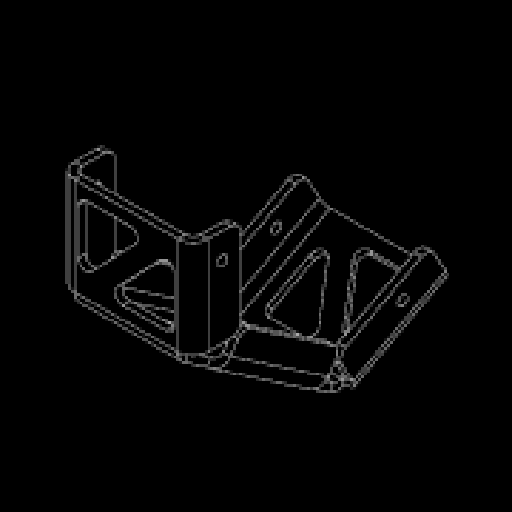
# Autodesk Inventor part: HipCoverTop
Saved by Autodesk Inventor 2025.2 (Build 292293000, 293)
## iProperties
Created: 2020-05-24
Part Number: HipCoverTop
Material: Generic
Document SubType Name: Sheet Metal
Designer: valer
Density: 1 g/cm^3
Sheet Metal Rule: Default
Appearance: Default
Author: valer
Autodesk Inventor part; units mm, degrees
ref_plane "YZ Plane" through (0, 0, 0) normal (1, 0, 0) x (0, 1, 0)
ref_plane "XZ Plane" through (0, 0, 0) normal (0, 1, 0) x (-1, 0, 0)
ref_plane "XY Plane" through (0, 0, 0) normal (0, 0, 1) x (1, 0, 0)
sketch "Base" plane through (0, 0, 0) normal (0, 0, 1) x (1, 0, 0)
  line L0 (0, 0) -> (44.58, 0)
  line L1 (44.58, 0) -> (44.58, -65.2018)
  line L2 (44.58, -65.2018) -> (0, -65.2018)
  line L3 (0, -65.2018) -> (0, 0)
  dimension "d0" = 65.2018
  dimension "d1" = 44.58
  measures "d0" distance of L2.end L0.start
  measures "d1" distance of L0.start L0.end
extrude "Plate1" add sketch "Base" along normal blind 5
sketch "Sketch2" plane through (5, 0, 5) normal (-1, 0, 0) x (0, -1, 0)
  line L0 (65.2018, 0) -> (0, 0)
  line L1 (0, 0) -> (0, -31.75)
  line L2 (0, -31.75) -> (65.2018, -31.75)
  line L3 (65.2018, -31.75) -> (65.2018, 0)
  constraints: 6 end point, 1 horizontal, 1 perpendicular, 1 vertical
edge flange "MountFeature" height 31.75 angle 90 thickness 5 bend radius 5 thickness toward (-1, 0, 0) relief straight relief width 5 relief depth 2.5 edges at (0, -32.6009, 0) wall of the first edge with corners at (5, -65.2018, 5) (5, 0, 5) (5, 0, -26.75) (5, -65.2018, -26.75)
bend "Bend1"
corner "Corner1"
mirror "MirrorFeature" about plane through (44.58, 0, 0) normal (1, 0, 0)
sketch "GenerativeCut1" plane through (0, 0, 5) normal (0, 0, 1) x (1, 0, 0)
  line L0 (12.7, -8.4667) -> (12.7, -56.7351)
  line L1 (12.7, -56.7351) -> (58.8832, -8.4667)
  line L2 (58.8832, -8.4667) -> (12.7, -8.4667)
  line L3 (79.16, 0) -> (10, 0) projected
  line L4 (30.2768, -56.7351) -> (76.46, -8.4667)
  line L5 (76.46, -8.4667) -> (76.46, -56.7351)
  line L6 (76.46, -56.7351) -> (30.2768, -56.7351)
  line L7 (58.8832, -8.4667) -> (76.46, -8.4667) construction
  line L8 (12.7, -56.7351) -> (30.2768, -56.7351) construction
  line L9 (0, -65.2018) -> (0, 0) projected
  line L10 (89.16, -65.2018) -> (89.16, 0) projected
  line L11 (79.16, -65.2018) -> (10, -65.2018) projected
  dimension "d23" = 8.4667
  dimension "d24" = 12.7
  dimension "d25" = 12.7
  dimension "d26" = 8.4667
  dimension "d27" = 12.7
  constraints: 16 end point, 2 parallel, 2 perpendicular, 1 collinear, 1 horizontal, 1 vertical
  measures "d23" distance between parallel lines of L3 L2
  measures "d24" distance between parallel lines of L9 L0
  measures "d25" distance between parallel lines of L5 L10
  measures "d26" distance between parallel lines of L11 L6
  measures "d27" distance between parallel lines of L4 L1
extrude "GenerativeCut1Feature" cut sketch "GenerativeCut1" against normal blind 25.4
fillet "GenerativeCut1FilletsFeature" radius 5.08 6 edges at (12.7, -8.4667, 2.5) (12.7, -56.7351, 2.5) (58.8832, -8.4667, 2.5) (76.46, -8.4667, 2.5) (30.2768, -56.7351, 2.5) (76.46, -56.7351, 2.5)
sketch "Sketch5" plane through (79.16, -69.3397, -2.1932) normal (0, -0.8275708, 0.5613614) x (1, 0, 0)
  line L0 (-69.16, 0) -> (0, 0)
  line L1 (0, 0) -> (0, 116.6197)
  line L2 (0, 116.6197) -> (-69.16, 116.6197)
  line L3 (-69.16, 116.6197) -> (-69.16, 0)
  constraints: 6 end point, 1 horizontal, 1 perpendicular, 1 vertical
edge flange "KneeFlangeFeature" height 121.92 angle 55.85 thickness 5 bend radius 5 thickness toward (0, -0.8275708, 0.5613614) relief straight relief width 5 relief depth 2.5 edges at (44.58, -65.2018, 5) wall of the first edge with corners at (10, -69.3397, -2.1932) (79.16, -69.3397, -2.1932) (79.16, -134.8054, -98.7042) (10, -134.8054, -98.7042)
bend "Bend2"
corner "Corner2"
sketch "Sketch6" plane through (10, -135.0807, -103.8615) normal (0, -0.8826196, -0.4700879) x (1, 0, 0)
  line L0 (69.16, 0) -> (0, 0)
  line L1 (0, 0) -> (0, -70.1688)
  line L2 (0, -70.1688) -> (69.16, -70.1688)
  line L3 (69.16, -70.1688) -> (69.16, 0)
  constraints: 6 end point, 1 horizontal, 1 perpendicular, 1 vertical
edge flange "KneeBottomFlangeFeature" height 76.2 angle 62.19 thickness 5 bend radius 5 thickness toward (0, -0.8826196, -0.4700879) relief straight relief width 5 relief depth 2.5 edges at (44.58, -134.8054, -98.7042) wall of the first edge with corners at (79.16, -135.0807, -103.8615) (10, -135.0807, -103.8615) (10, -102.0952, -165.7938) (79.16, -102.0952, -165.7938)
bend "Bend3"
corner "Corner3"
sketch "Sketch8" plane through (5, -130.6676, -101.511) normal (-1, 0, 0) x (0, -1, 0)
  line L0 (-32.9855, -61.9324) -> (0, 0)
  line L1 (0, 0) -> (-19.197, 10.2244)
  line L2 (-19.197, 10.2244) -> (-52.1825, -51.708)
  line L3 (-52.1825, -51.708) -> (-32.9855, -61.9324)
  constraints: 6 end point, 1 perpendicular, 2 other
edge flange "KneeBottomSidesFeature" height 31.75 angle 90 thickness 5 bend radius 5 thickness toward (-1, 0, 0) relief straight relief width 5 relief depth 2.5 corner gap 5 corner form 0 edges at (10, -118.5879, -134.8277) (79.16, -118.5879, -134.8277) wall of the first edge with corners at (5, -97.6821, -163.4434) (5, -130.6676, -101.511) (5, -111.4706, -91.2866) (5, -78.4851, -153.219)
bend "Bend4"
corner "Corner4"
fillet "OutsideFilletsFeature" radius 6.35 8 edges at (2.5, -65.2018, -26.75) (2.5, 0, -26.75) (2.5, -111.4706, -91.2866) (86.66, -78.4851, -153.219) (2.5, -78.4851, -153.219) (86.66, -111.4706, -91.2866) (86.66, -65.2018, -26.75) (86.66, 0, -26.75)
sketch "Sketch10" plane through (10, -73.4775, 0.6136) normal (0, -0.8275708, 0.5613614) x (1, 0, 0)
  line L0 (-5, -15.5299) -> (-10, -15.5299) projected
  line L1 (-5, -99.6109) -> (-10, -99.6109) projected
  line L2 (-10, -18.0699) -> (0, -18.0699)
  line L3 (0, -18.0699) -> (0, -97.0709)
  line L4 (0, -97.0709) -> (-10, -97.0709)
  line L5 (-10, -97.0709) -> (-10, -18.0699)
  line L6 (-10, 0) -> (-10, -12.7446) projected
  line L7 (0, 0) -> (0, -116.6197) projected
  point P0 (-10, 40.7396)
  dimension "d65" = 2.54
  dimension "d66" = 2.54
  constraints: 8 end point, 2 collinear, 2 parallel, 1 horizontal, 1 perpendicular
  measures "d65" distance between parallel lines of L0 L2
  measures "d66" distance between parallel lines of L1 L4
sheet face with bend "SideFlangeBaseFeature" sketch "Sketch10" thickness 5 toward (0, 0.8275708, -0.5613614) bend radius 5 relief straight relief width 5 relief depth 2.5
bend "Bend5"
sketch "Sketch11" plane through (5, -83.6213, -14.3405) normal (-1, 0, 0) x (0, -1, 0)
  line L0 (44.3481, -65.3789) -> (0, 0)
  line L1 (0, 0) -> (-21.0203, -14.2586)
  line L2 (-21.0203, -14.2586) -> (23.3278, -79.6375)
  line L3 (23.3278, -79.6375) -> (44.3481, -65.3789)
  constraints: 6 end point, 1 perpendicular, 2 other
edge flange "SideFlangeFeature" height 25.4 angle 90 thickness 5 bend radius 5 thickness toward (-1, 0, 0) relief straight relief width 5 relief depth 2.5 edges at (0, -101.6575, -49.8368) wall of the first edge with corners at (5, -127.9694, -79.7194) (5, -83.6213, -14.3405) (5, -62.601, -28.5991) (5, -106.9491, -93.978)
bend "Bend6"
corner "Corner5"
ref_plane "MiddlePlane" through (44.58, -97.6821, -163.4434) normal (-1, 0, 0) x (0, -0.4700879, 0.8826196)
mirror "SideFlangeMirrorFeature" about plane through (44.58, -97.6821, -163.4434) normal (-1, 0, 0) of "SideFlangeFeature"
fillet "SideFlangeFilletsFeature" radius 6.35 4 edges at (2.5, -106.9491, -93.978) (86.66, -106.9491, -93.978) (2.5, -62.601, -28.5991) (86.66, -62.601, -28.5991)
sketch "Rais" plane through (10, -73.4775, 0.6136) normal (0, -0.8275708, 0.5613614) x (1, 0, 0)
  line L0 (69.16, 0) -> (0, 0) construction
  line L1 (0, -116.6197) -> (69.16, -116.6197) construction
  line L2 (0, 0) -> (69.16, 0) construction
  line L3 (34.58, 0) -> (34.58, -116.6197) construction
  line L4 (0, -116.6197) -> (69.16, -116.6197) construction
  line L5 (26.3701, -42.5901) -> (17.3899, -33.6099) construction
  line L6 (24.1251, -44.8352) -> (15.1448, -35.8549)
  line L7 (19.6349, -31.3648) -> (28.6152, -40.3451)
  arc A0 (24.1251, -44.8352) -> (28.6152, -40.3451) centre (26.3701, -42.5901) ccw
  arc A1 (19.6349, -31.3648) -> (15.1448, -35.8549) centre (17.3899, -33.6099) ccw
  line L8 (0, -18.0699) -> (0, -97.0709) construction
  line L9 (0, -57.5704) -> (69.16, -57.5704) construction
  line L10 (69.16, -97.0709) -> (69.16, -18.0699) construction
  line L11 (45.0349, -44.8352) -> (54.0152, -35.8549)
  line L12 (49.5251, -31.3648) -> (40.5448, -40.3451)
  arc A2 (40.5448, -40.3451) -> (45.0349, -44.8352) centre (42.7899, -42.5901) ccw
  arc A3 (54.0152, -35.8549) -> (49.5251, -31.3648) centre (51.7701, -33.6099) ccw
  line L13 (24.1251, -70.3057) -> (15.1448, -79.2859)
  line L14 (19.6349, -83.7761) -> (28.6152, -74.7958)
  arc A4 (28.6152, -74.7958) -> (24.1251, -70.3057) centre (26.3701, -72.5507) ccw
  arc A5 (15.1448, -79.2859) -> (19.6349, -83.7761) centre (17.3899, -81.531) ccw
  line L15 (45.0349, -70.3057) -> (54.0152, -79.2859)
  arc A6 (49.5251, -83.7761) -> (54.0152, -79.2859) centre (51.7701, -81.531) ccw
  line L16 (49.5251, -83.7761) -> (40.5448, -74.7958)
  arc A7 (45.0349, -70.3057) -> (40.5448, -74.7958) centre (42.7899, -72.5507) ccw
  point P0 (-10, 40.7396)
  point P1 (21.88, -38.1)
  dimension "d101" = 3.175
  dimension "d102" = 12.7
  dimension "d103" = 12.7
  dimension "d104" = 38.1
  dimension "d105" = 45
  constraints: 24 end point, 18 symmetric about line, 16 point on circle, 8 centre point, 5 midpoint, 4 tangent, 1 parallel, 6 other
  measures "d101" radius of A1
  measures "d102" distance from line of L3 point (21.88, -38.1)
  measures "d103" distance of L5.start L5.end
  measures "d104" distance from line of L0 point (21.88, -38.1)
  measures "d105" angle of L3 L5
extrude "RailsFeature" cut sketch "Rais" against normal blind 25.4
sketch "GenerativeCut2" plane through (10, -139.4938, -106.2119) normal (0, -0.8826196, -0.4700879) x (1, 0, 0)
  line L0 (8.4667, -8.4667) -> (8.4667, -61.7021)
  line L1 (8.4667, -61.7021) -> (45.2558, -8.4667)
  line L2 (45.2558, -8.4667) -> (8.4667, -8.4667)
  line L3 (23.9042, -61.7021) -> (60.6933, -8.4667)
  line L4 (60.6933, -8.4667) -> (60.6933, -61.7021)
  line L5 (60.6933, -61.7021) -> (23.9042, -61.7021)
  line L6 (45.2558, -8.4667) -> (60.6933, -8.4667) construction
  line L7 (8.4667, -61.7021) -> (23.9042, -61.7021) construction
  line L8 (69.16, 0) -> (0, 0) projected
  line L9 (0, -70.1688) -> (0, 0) projected
  line L10 (69.16, -70.1688) -> (0, -70.1688) projected
  line L11 (69.16, 0) -> (69.16, -70.1688) projected
  point P0 (-10, 28.1704)
  dimension "d124" = 12.7
  dimension "d125" = 8.4667
  dimension "d126" = 8.4667
  dimension "d127" = 8.4667
  dimension "d128" = 8.4667
  constraints: 16 end point, 2 perpendicular, 1 collinear, 1 horizontal, 1 parallel, 1 vertical
  measures "d124" distance between parallel lines of L3 L1
  measures "d125" distance between parallel lines of L8 L2
  measures "d126" distance between parallel lines of L9 L0
  measures "d127" distance between parallel lines of L11 L4
  measures "d128" distance between parallel lines of L10 L5
extrude "GenerativeCut2Feature" cut sketch "GenerativeCut2" against normal blind 25.4 contours L2 L1 L0 | L3 L4 L5
fillet "GenerativeCut2FilletsFeature" radius 5.08 6 edges at (18.4667, -133.3072, -112.5095) (55.2558, -133.3072, -112.5095) (18.4667, -108.2818, -159.4962) (33.9042, -108.2818, -159.4962) (70.6933, -133.3072, -112.5095) (70.6933, -108.2818, -159.4962)
sketch "Sketch17" plane through (0, -97.6821, -163.4434) normal (-1, 0, 0) x (0, -0.4700879, 0.8826196)
  line L0 (90.5478, 141.3686) -> (91.5775, 154.0268) construction
  arc A0 (90.5478, 141.3686) -> (96.8769, 140.8537) centre (93.7123, 141.1111) ccw construction
  line L1 (97.9065, 153.5119) -> (96.8769, 140.8537) construction
  arc A1 (97.9065, 153.5119) -> (91.5775, 154.0268) centre (94.742, 153.7693) ccw construction
  line L2 (106.5897, 106.2825) -> (119.2731, 106.9319) construction
  arc A2 (106.5897, 106.2825) -> (106.9144, 99.9408) centre (106.752, 103.1116) ccw construction
  line L3 (119.5978, 100.5902) -> (106.9144, 99.9408) construction
  arc A3 (119.5978, 100.5902) -> (119.2731, 106.9319) centre (119.4354, 103.761) ccw construction
  arc A4 (68.1033, 17.0403) -> (62.0892, 15.0025) centre (65.0963, 16.0214) ccw construction
  line L4 (66.1647, 2.9742) -> (62.0892, 15.0025) construction
  arc A5 (66.1647, 2.9742) -> (72.1789, 5.012) centre (69.1718, 3.9931) ccw construction
  line L5 (68.1033, 17.0403) -> (72.1789, 5.012) construction
  line L6 (22.4017, 5.2914) -> (24.4573, 17.8239) construction
  arc A6 (30.7236, 16.7961) -> (24.4573, 17.8239) centre (27.5904, 17.31) ccw construction
  line L7 (30.7236, 16.7961) -> (28.668, 4.2636) construction
  arc A7 (22.4017, 5.2914) -> (28.668, 4.2636) centre (25.5348, 4.7775) ccw construction
  circle A8 centre (93.7123, 141.1111) radius 3.175
  line L8 (27.5904, 17.31) -> (25.5348, 4.7775) construction
  circle A9 centre (26.5626, 11.0437) radius 3.175
  line L9 (119.4354, 103.761) -> (106.752, 103.1116) construction
  line L10 (65.0963, 16.0214) -> (69.1718, 3.9931) construction
  point P0 (98.3392, 163.0489)
  dimension "d134" = 6.35
  dimension "d135" = 6.35
  constraints: 6 end point, 1 centre point, 1 coincident, 1 midpoint, 1 tangent, 3 other
  measures "d135" diameter of A9
extrude "Cut1" cut sketch "Sketch17" against normal through all
equation "\"d25\" = d24"
equation "\"d26\" = d23"
equation "\"d27\" = d24"
equation "\"d124\" = d121"
equation "\"d132\" = Thickness"
equation "\"d2\" = Thickness"
equation "\"d3\" = BendReliefWidth"
equation "\"d4\" = BendReliefDepth"
equation "\"d5\" = MinimumRemnant"
equation "\"d6\" = TransitionRadius"
equation "\"d9\" = BendRadius"
equation "\"d10\" = CornerReliefSize"
equation "\"d11\" = GapSize"
equation "\"d12\" = JacobiRadiusSize"
equation "\"d31\" = BendReliefWidth"
equation "\"d32\" = BendReliefDepth"
equation "\"d33\" = MinimumRemnant"
equation "\"d34\" = TransitionRadius"
equation "\"d37\" = BendRadius"
equation "\"d38\" = CornerReliefSize"
equation "\"d39\" = GapSize"
equation "\"d40\" = JacobiRadiusSize"
equation "\"d41\" = BendReliefWidth"
equation "\"d42\" = BendReliefDepth"
equation "\"d43\" = MinimumRemnant"
equation "\"d44\" = TransitionRadius"
equation "\"d47\" = BendRadius"
equation "\"d48\" = CornerReliefSize"
equation "\"d49\" = GapSize"
equation "\"d50\" = JacobiRadiusSize"
equation "\"d51\" = BendReliefWidth"
equation "\"d52\" = BendReliefDepth"
equation "\"d53\" = MinimumRemnant"
equation "\"d54\" = TransitionRadius"
equation "\"d57\" = BendRadius"
equation "\"d58\" = CornerReliefSize"
equation "\"d59\" = GapSize"
equation "\"d60\" = JacobiRadiusSize"
equation "\"d66\" = d65"
equation "\"d67\" = BendRadius"
equation "\"d68\" = BendReliefWidth"
equation "\"d70\" = MinimumRemnant"
equation "\"d69\" = BendReliefDepth"
equation "\"d71\" = TransitionRadius"
equation "\"d72\" = BendReliefWidth"
equation "\"d73\" = BendReliefDepth"
equation "\"d74\" = MinimumRemnant"
equation "\"d75\" = TransitionRadius"
equation "\"d78\" = BendRadius"
equation "\"d79\" = CornerReliefSize"
equation "\"d80\" = GapSize"
equation "\"d81\" = JacobiRadiusSize"
equation "\"BendRadius\" = Thickness"
equation "\"BendReliefWidth\" = Thickness"
equation "\"BendReliefDepth\" = 0.5 * Thickness"
equation "\"TransitionRadius\" = BendRadius"
equation "\"JacobiRadiusSize\" = BendRadius"
equation "\"GapSize\" = Thickness"
equation "\"d121\" = 12.7"
equation "\"Thickness\" = 5"
equation "\"MinimumRemnant\" = 10"
equation "\"CornerReliefSize\" = 20"
body "Solid1"
